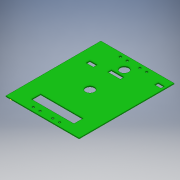
# Autodesk Inventor part: Aquila-2018-Under
Saved by Autodesk Inventor 2018 (Build 220112000, 112)
## iProperties
Created: 2018-08-01
Part Number: Aquila-2018-Under
Material: 一般
Document SubType Name: Modeling
Designer: shun2
Density: 1 g/cm^3
Appearance: 濃い緑
Author: shun2
Autodesk Inventor part; units mm, degrees
ref_plane "YZ Plane" through (0, 0, 0) normal (1, 0, 0) x (0, 1, 0)
ref_plane "XZ Plane" through (0, 0, 0) normal (0, 1, 0) x (-1, 0, 0)
ref_plane "XY Plane" through (0, 0, 0) normal (0, 0, 1) x (1, 0, 0)
sketch "スケッチ4" plane through (0, 0, 0) normal (0, 0, 1) x (1, 0, 0)
  circle A0 centre (127.58, 175.805) radius 0.35
  circle A1 centre (23.4696, 144.78) radius 0.6604
  circle A2 centre (18.4404, 144.78) radius 0.6604
  circle A3 centre (100.9396, 26.035) radius 0.6604
  circle A4 centre (95.9104, 26.035) radius 0.6604
  circle A5 centre (63.105, 150.54) radius 0.6
  circle A6 centre (65.645, 150.54) radius 0.6
  circle A7 centre (68.185, 150.54) radius 0.6
  circle A8 centre (89.59, 26.34) radius 0.6
  circle A9 centre (87.05, 26.34) radius 0.6
  circle A10 centre (84.51, 26.34) radius 0.6
  circle A11 centre (62.96, 25.555) radius 0.508
  circle A12 centre (65.5, 25.555) radius 0.508
  circle A13 centre (68.04, 25.555) radius 0.508
  circle A14 centre (70.58, 25.555) radius 0.508
  circle A15 centre (60.42, 25.555) radius 0.508
  circle A16 centre (75.66, 25.555) radius 0.508
  circle A17 centre (57.88, 25.555) radius 0.508
  circle A18 centre (55.34, 25.555) radius 0.508
  circle A19 centre (78.2, 25.555) radius 0.508
  circle A20 centre (52.8, 25.555) radius 0.508
  circle A21 centre (73.12, 25.555) radius 0.508
  circle A22 centre (50.26, 25.555) radius 0.508
  circle A23 centre (47.72, 25.555) radius 0.508
  circle A24 centre (129.08, 175.805) radius 0.35
  circle A25 centre (130.58, 175.805) radius 0.35
  circle A26 centre (132.08, 175.805) radius 0.35
  circle A27 centre (133.58, 175.805) radius 0.35
  circle A28 centre (124.58, 175.805) radius 0.35
  circle A29 centre (126.08, 175.805) radius 0.35
  circle A30 centre (38, 8) radius 2.15
  circle A31 centre (52, 8) radius 2.15
  circle A32 centre (92, 8) radius 2.15
  circle A33 centre (92, 186.7239) radius 2.15
  circle A34 centre (78, 8) radius 2.15
  circle A35 centre (52, 186.7215) radius 2.15
  circle A36 centre (38, 186.7239) radius 2.15
  circle A37 centre (78, 186.7215) radius 2.15
  line L0 (58.919, 174.3601) -> (58.7286, 174.1804)
  line L1 (58.7286, 174.1804) -> (58.5435, 173.9953)
  line L2 (58.5435, 173.9953) -> (58.3638, 173.8049)
  line L3 (58.3638, 173.8049) -> (58.1897, 173.6093)
  line L4 (58.1897, 173.6093) -> (58.0215, 173.4087)
  line L5 (58.0215, 173.4087) -> (57.8591, 173.2034)
  line L6 (57.8591, 173.2034) -> (57.7027, 172.9933)
  line L7 (57.7027, 172.9933) -> (57.5525, 172.7789)
  line L8 (57.5525, 172.7789) -> (57.4087, 172.5601)
  line L9 (57.4087, 172.5601) -> (57.2712, 172.3373)
  line L10 (57.2712, 172.3373) -> (57.1403, 172.1105)
  line L11 (57.1403, 172.1105) -> (57.0161, 171.8801)
  line L12 (57.0161, 171.8801) -> (56.8986, 171.6461)
  line L13 (56.8986, 171.6461) -> (56.7879, 171.4088)
  line L14 (56.7879, 171.4088) -> (56.6842, 171.1684)
  line L15 (56.6842, 171.1684) -> (56.5875, 170.9251)
  line L16 (56.5875, 170.9251) -> (56.498, 170.6791)
  line L17 (56.498, 170.6791) -> (56.4156, 170.4306)
  line L18 (56.4156, 170.4306) -> (56.3406, 170.1797)
  line L19 (56.3406, 170.1797) -> (56.2728, 169.9268)
  line L20 (56.2728, 169.9268) -> (56.2124, 169.6721)
  line L21 (56.2124, 169.6721) -> (56.1595, 169.4157)
  line L22 (56.1595, 169.4157) -> (56.114, 169.1578)
  line L23 (56.114, 169.1578) -> (56.0761, 168.8988)
  line L24 (56.0761, 168.8988) -> (56.0457, 168.6387)
  line L25 (56.0457, 168.6387) -> (56.0228, 168.3779)
  line L26 (56.0228, 168.3779) -> (56.0076, 168.1165)
  line L27 (56.0076, 168.1165) -> (56, 167.8548)
  line L28 (56, 167.8548) -> (56, 167.593)
  line L29 (56, 167.593) -> (56.0076, 167.3313)
  line L30 (56.0076, 167.3313) -> (56.0228, 167.0699)
  line L31 (56.0228, 167.0699) -> (56.0457, 166.8091)
  line L32 (56.0457, 166.8091) -> (56.0761, 166.5491)
  line L33 (56.0761, 166.5491) -> (56.114, 166.29)
  line L34 (56.114, 166.29) -> (56.1595, 166.0322)
  line L35 (56.1595, 166.0322) -> (56.2124, 165.7758)
  line L36 (56.2124, 165.7758) -> (56.2728, 165.521)
  line L37 (56.2728, 165.521) -> (56.3406, 165.2681)
  line L38 (56.3406, 165.2681) -> (56.4156, 165.0173)
  line L39 (56.4156, 165.0173) -> (56.498, 164.7688)
  line L40 (56.498, 164.7688) -> (56.5875, 164.5227)
  line L41 (56.5875, 164.5227) -> (56.6842, 164.2794)
  line L42 (56.6842, 164.2794) -> (56.7879, 164.039)
  line L43 (56.7879, 164.039) -> (56.8986, 163.8017)
  line L44 (56.8986, 163.8017) -> (57.0161, 163.5677)
  line L45 (57.0161, 163.5677) -> (57.1403, 163.3373)
  line L46 (57.1403, 163.3373) -> (57.2712, 163.1105)
  line L47 (57.2712, 163.1105) -> (57.4087, 162.8877)
  line L48 (57.4087, 162.8877) -> (57.5525, 162.669)
  line L49 (57.5525, 162.669) -> (57.7027, 162.4545)
  line L50 (57.7027, 162.4545) -> (57.8591, 162.2445)
  line L51 (57.8591, 162.2445) -> (58.0215, 162.0391)
  line L52 (58.0215, 162.0391) -> (58.1897, 161.8385)
  line L53 (58.1897, 161.8385) -> (58.3638, 161.643)
  line L54 (58.3638, 161.643) -> (58.5435, 161.4525)
  line L55 (58.5435, 161.4525) -> (58.7286, 161.2674)
  line L56 (58.7286, 161.2674) -> (58.919, 161.0877)
  line L57 (58.919, 161.0877) -> (59.1146, 160.9137)
  line L58 (59.1146, 160.9137) -> (59.3152, 160.7454)
  line L59 (59.3152, 160.7454) -> (59.5206, 160.583)
  line L60 (59.5206, 160.583) -> (59.7306, 160.4266)
  line L61 (59.7306, 160.4266) -> (59.945, 160.2765)
  line L62 (59.945, 160.2765) -> (60.1638, 160.1326)
  line L63 (60.1638, 160.1326) -> (60.3866, 159.9951)
  line L64 (60.3866, 159.9951) -> (60.6134, 159.8642)
  line L65 (60.6134, 159.8642) -> (60.8438, 159.74)
  line L66 (60.8438, 159.74) -> (61.0778, 159.6225)
  line L67 (61.0778, 159.6225) -> (61.3151, 159.5118)
  line L68 (69.1562, 89.378) -> (69.3866, 89.5023)
  line L69 (61.5555, 159.4081) -> (61.7988, 159.3115)
  line L70 (61.7988, 159.3115) -> (62.0448, 159.2219)
  line L71 (62.0448, 159.2219) -> (62.2934, 159.1396)
  line L72 (62.2934, 159.1396) -> (62.5442, 159.0645)
  line L73 (62.5442, 159.0645) -> (62.7971, 158.9967)
  line L74 (62.7971, 158.9967) -> (63.0518, 158.9363)
  line L75 (63.0518, 158.9363) -> (63.3082, 158.8834)
  line L76 (63.3082, 158.8834) -> (63.5661, 158.8379)
  line L77 (63.5661, 158.8379) -> (63.8251, 158.8)
  line L78 (63.8251, 158.8) -> (64.0852, 158.7696)
  line L79 (64.0852, 158.7696) -> (64.346, 158.7468)
  line L80 (64.346, 158.7468) -> (64.6074, 158.7315)
  line L81 (64.6074, 158.7315) -> (64.8691, 158.7239)
  line L82 (64.8691, 158.7239) -> (65.1309, 158.7239)
  line L83 (65.1309, 158.7239) -> (65.3926, 158.7315)
  line L84 (65.3926, 158.7315) -> (65.654, 158.7468)
  line L85 (65.654, 158.7468) -> (65.9148, 158.7696)
  line L86 (65.9148, 158.7696) -> (66.1749, 158.8)
  line L87 (66.1749, 158.8) -> (66.4339, 158.8379)
  line L88 (66.4339, 158.8379) -> (66.6918, 158.8834)
  line L89 (66.6918, 158.8834) -> (66.9482, 158.9363)
  line L90 (66.9482, 158.9363) -> (67.2029, 158.9967)
  line L91 (67.2029, 158.9967) -> (67.4558, 159.0645)
  line L92 (67.4558, 159.0645) -> (67.7066, 159.1396)
  line L93 (67.7066, 159.1396) -> (67.9552, 159.2219)
  line L94 (67.9552, 159.2219) -> (68.2012, 159.3115)
  line L95 (68.2012, 159.3115) -> (68.4445, 159.4081)
  line L96 (68.4445, 159.4081) -> (68.6849, 159.5118)
  line L97 (68.6849, 159.5118) -> (68.9222, 159.6225)
  line L98 (68.9222, 159.6225) -> (69.1562, 159.74)
  line L99 (69.1562, 159.74) -> (69.3866, 159.8642)
  line L100 (69.3866, 159.8642) -> (69.6134, 159.9951)
  line L101 (69.6134, 159.9951) -> (69.8362, 160.1326)
  line L102 (69.8362, 160.1326) -> (70.055, 160.2765)
  line L103 (70.055, 160.2765) -> (70.2694, 160.4266)
  line L104 (70.2694, 160.4266) -> (70.4794, 160.583)
  line L105 (70.4794, 160.583) -> (70.6848, 160.7454)
  line L106 (70.6848, 160.7454) -> (70.8854, 160.9137)
  line L107 (70.8854, 160.9137) -> (71.081, 161.0877)
  line L108 (71.081, 161.0877) -> (71.2714, 161.2674)
  line L109 (71.2714, 161.2674) -> (71.4565, 161.4525)
  line L110 (71.4565, 161.4525) -> (71.6362, 161.643)
  line L111 (71.6362, 161.643) -> (71.8103, 161.8385)
  line L112 (71.8103, 161.8385) -> (71.9785, 162.0391)
  line L113 (71.9785, 162.0391) -> (72.1409, 162.2445)
  line L114 (72.1409, 162.2445) -> (72.2973, 162.4545)
  line L115 (72.2973, 162.4545) -> (72.4475, 162.669)
  line L116 (72.4475, 162.669) -> (72.5913, 162.8877)
  line L117 (72.5913, 162.8877) -> (72.7288, 163.1105)
  line L118 (72.7288, 163.1105) -> (72.8597, 163.3373)
  line L119 (72.8597, 163.3373) -> (72.9839, 163.5677)
  line L120 (72.9839, 163.5677) -> (73.1014, 163.8017)
  line L121 (73.1014, 163.8017) -> (73.2121, 164.039)
  line L122 (73.2121, 164.039) -> (73.3158, 164.2794)
  line L123 (73.3158, 164.2794) -> (73.4125, 164.5227)
  line L124 (73.4125, 164.5227) -> (73.502, 164.7688)
  line L125 (73.502, 164.7688) -> (73.5844, 165.0173)
  line L126 (73.5844, 165.0173) -> (73.6595, 165.2681)
  line L127 (73.6595, 165.2681) -> (73.7272, 165.521)
  line L128 (73.7272, 165.521) -> (73.7876, 165.7758)
  line L129 (73.7876, 165.7758) -> (73.8405, 166.0322)
  line L130 (73.8405, 166.0322) -> (73.886, 166.29)
  line L131 (73.886, 166.29) -> (73.9239, 166.5491)
  line L132 (73.9239, 166.5491) -> (73.9543, 166.8091)
  line L133 (73.9543, 166.8091) -> (73.9772, 167.0699)
  line L134 (73.9772, 167.0699) -> (73.9924, 167.3313)
  line L135 (73.9924, 167.3313) -> (74, 167.593)
  line L136 (57.7027, 102.6314) -> (57.5525, 102.4169)
  line L137 (74, 97.2311) -> (74, 97.4929)
  line L138 (74, 97.4929) -> (73.9924, 97.7546)
  line L139 (73.9924, 97.7546) -> (73.9772, 98.016)
  line L140 (73.9772, 98.016) -> (73.9543, 98.2768)
  line L141 (73.9543, 98.2768) -> (73.9239, 98.5368)
  line L142 (73.9239, 98.5368) -> (73.886, 98.7959)
  line L143 (73.886, 98.7959) -> (73.8405, 99.0537)
  line L144 (73.8405, 99.0537) -> (73.7876, 99.3101)
  line L145 (73.7876, 99.3101) -> (73.7272, 99.5649)
  line L146 (73.7272, 99.5649) -> (73.6595, 99.8178)
  line L147 (73.6595, 99.8178) -> (73.5844, 100.0686)
  line L148 (73.5844, 100.0686) -> (73.502, 100.3171)
  line L149 (73.502, 100.3171) -> (73.4125, 100.5632)
  line L150 (73.4125, 100.5632) -> (73.3158, 100.8065)
  line L151 (73.3158, 100.8065) -> (73.2121, 101.0469)
  line L152 (73.2121, 101.0469) -> (73.1014, 101.2842)
  line L153 (73.1014, 101.2842) -> (72.9839, 101.5181)
  line L154 (61.3151, 159.5118) -> (61.5555, 159.4081)
  line L155 (72.9839, 101.5181) -> (72.8597, 101.7486)
  line L156 (72.8597, 101.7486) -> (72.7288, 101.9753)
  line L157 (72.7288, 101.9753) -> (72.5913, 102.1982)
  line L158 (72.5913, 102.1982) -> (72.4475, 102.4169)
  line L159 (72.4475, 102.4169) -> (72.2973, 102.6314)
  line L160 (72.2973, 102.6314) -> (72.1409, 102.8414)
  line L161 (72.1409, 102.8414) -> (71.9785, 103.0468)
  line L162 (71.9785, 103.0468) -> (71.8103, 103.2473)
  line L163 (71.8103, 103.2473) -> (71.6362, 103.4429)
  line L164 (71.6362, 103.4429) -> (71.4565, 103.6334)
  line L165 (71.4565, 103.6334) -> (71.2714, 103.8185)
  line L166 (71.2714, 103.8185) -> (71.081, 103.9982)
  line L167 (71.081, 103.9982) -> (70.8854, 104.1722)
  line L168 (70.8854, 104.1722) -> (70.6848, 104.3405)
  line L169 (70.6848, 104.3405) -> (70.4794, 104.5029)
  line L170 (70.4794, 104.5029) -> (70.2694, 104.6592)
  line L171 (70.2694, 104.6592) -> (70.055, 104.8094)
  line L172 (70.055, 104.8094) -> (69.8362, 104.9533)
  line L173 (69.8362, 104.9533) -> (69.6134, 105.0907)
  line L174 (69.6134, 105.0907) -> (69.3866, 105.2216)
  line L175 (69.3866, 105.2216) -> (69.1562, 105.3459)
  line L176 (69.1562, 105.3459) -> (68.9222, 105.4634)
  line L177 (68.9222, 105.4634) -> (68.6849, 105.5741)
  line L178 (68.6849, 105.5741) -> (68.4445, 105.6778)
  line L179 (68.4445, 105.6778) -> (68.2012, 105.7744)
  line L180 (68.2012, 105.7744) -> (67.9552, 105.864)
  line L181 (67.9552, 105.864) -> (67.7066, 105.9463)
  line L182 (67.7066, 105.9463) -> (67.4558, 106.0214)
  line L183 (67.4558, 106.0214) -> (67.2029, 106.0892)
  line L184 (67.2029, 106.0892) -> (66.9482, 106.1496)
  line L185 (66.9482, 106.1496) -> (66.6918, 106.2025)
  line L186 (66.6918, 106.2025) -> (66.4339, 106.248)
  line L187 (66.4339, 106.248) -> (66.1749, 106.2859)
  line L188 (66.1749, 106.2859) -> (65.9148, 106.3163)
  line L189 (65.9148, 106.3163) -> (65.654, 106.3391)
  line L190 (65.654, 106.3391) -> (65.3926, 106.3543)
  line L191 (65.3926, 106.3543) -> (65.1309, 106.362)
  line L192 (65.1309, 106.362) -> (64.8691, 106.362)
  line L193 (64.8691, 106.362) -> (64.6074, 106.3543)
  line L194 (64.6074, 106.3543) -> (64.346, 106.3391)
  line L195 (64.346, 106.3391) -> (64.0852, 106.3163)
  line L196 (64.0852, 106.3163) -> (63.8251, 106.2859)
  line L197 (63.8251, 106.2859) -> (63.5661, 106.248)
  line L198 (63.5661, 106.248) -> (63.3082, 106.2025)
  line L199 (63.3082, 106.2025) -> (63.0518, 106.1496)
  line L200 (63.0518, 106.1496) -> (62.7971, 106.0892)
  line L201 (62.7971, 106.0892) -> (62.5442, 106.0214)
  line L202 (62.5442, 106.0214) -> (62.2934, 105.9463)
  line L203 (62.2934, 105.9463) -> (62.0448, 105.864)
  line L204 (62.0448, 105.864) -> (61.7988, 105.7744)
  line L205 (61.7988, 105.7744) -> (61.5555, 105.6778)
  line L206 (61.5555, 105.6778) -> (61.3151, 105.5741)
  line L207 (61.3151, 105.5741) -> (61.0778, 105.4634)
  line L208 (61.0778, 105.4634) -> (60.8438, 105.3459)
  line L209 (60.8438, 105.3459) -> (60.6134, 105.2216)
  line L210 (60.6134, 105.2216) -> (60.3866, 105.0907)
  line L211 (60.3866, 105.0907) -> (60.1638, 104.9533)
  line L212 (60.1638, 104.9533) -> (59.945, 104.8094)
  line L213 (59.945, 104.8094) -> (59.7306, 104.6592)
  line L214 (59.7306, 104.6592) -> (59.5206, 104.5029)
  line L215 (59.5206, 104.5029) -> (59.3152, 104.3405)
  line L216 (59.3152, 104.3405) -> (59.1146, 104.1722)
  line L217 (59.1146, 104.1722) -> (58.919, 103.9982)
  line L218 (58.919, 103.9982) -> (58.7286, 103.8185)
  line L219 (58.7286, 103.8185) -> (58.5435, 103.6334)
  line L220 (58.5435, 103.6334) -> (58.3638, 103.4429)
  line L221 (58.3638, 103.4429) -> (58.1897, 103.2473)
  line L222 (58.1897, 103.2473) -> (58.0215, 103.0468)
  line L223 (58.0215, 103.0468) -> (57.8591, 102.8414)
  line L224 (57.8591, 102.8414) -> (57.7027, 102.6314)
  line L225 (57.5525, 102.4169) -> (57.4087, 102.1982)
  line L226 (57.4087, 102.1982) -> (57.2712, 101.9753)
  line L227 (57.2712, 101.9753) -> (57.1403, 101.7486)
  line L228 (57.1403, 101.7486) -> (57.0161, 101.5181)
  line L229 (57.0161, 101.5181) -> (56.8986, 101.2842)
  line L230 (56.8986, 101.2842) -> (56.7879, 101.0469)
  line L231 (56.7879, 101.0469) -> (56.6842, 100.8065)
  line L232 (56.6842, 100.8065) -> (56.5875, 100.5632)
  line L233 (56.5875, 100.5632) -> (56.498, 100.3171)
  line L234 (56.498, 100.3171) -> (56.4156, 100.0686)
  line L235 (56.4156, 100.0686) -> (56.3406, 99.8178)
  line L236 (56.3406, 99.8178) -> (56.2728, 99.5649)
  line L237 (56.2728, 99.5649) -> (56.2124, 99.3101)
  line L238 (56.2124, 99.3101) -> (56.1595, 99.0537)
  line L239 (56.1595, 99.0537) -> (56.114, 98.7959)
  line L240 (56.114, 98.7959) -> (56.0761, 98.5368)
  line L241 (56.0761, 98.5368) -> (56.0457, 98.2768)
  line L242 (56.0457, 98.2768) -> (56.0228, 98.016)
  line L243 (56.0228, 98.016) -> (56.0076, 97.7546)
  line L244 (56.0076, 97.7546) -> (56, 97.4929)
  line L245 (56, 97.4929) -> (56, 97.2311)
  line L246 (56, 97.2311) -> (56.0076, 96.9693)
  line L247 (56.0076, 96.9693) -> (56.0228, 96.708)
  line L248 (56.0228, 96.708) -> (56.0457, 96.4471)
  line L249 (56.0457, 96.4471) -> (56.0761, 96.1871)
  line L250 (56.0761, 96.1871) -> (56.114, 95.928)
  line L251 (56.114, 95.928) -> (56.1595, 95.6702)
  line L252 (56.1595, 95.6702) -> (56.2124, 95.4138)
  line L253 (56.2124, 95.4138) -> (56.2728, 95.159)
  line L254 (56.2728, 95.159) -> (56.3406, 94.9061)
  line L255 (56.3406, 94.9061) -> (56.4156, 94.6553)
  line L256 (56.4156, 94.6553) -> (56.498, 94.4068)
  line L257 (56.498, 94.4068) -> (56.5875, 94.1608)
  line L258 (56.5875, 94.1608) -> (56.6842, 93.9174)
  line L259 (56.6842, 93.9174) -> (56.7879, 93.677)
  line L260 (56.7879, 93.677) -> (56.8986, 93.4398)
  line L261 (56.8986, 93.4398) -> (57.0161, 93.2058)
  line L262 (57.0161, 93.2058) -> (57.1403, 92.9753)
  line L263 (57.1403, 92.9753) -> (57.2712, 92.7486)
  line L264 (57.2712, 92.7486) -> (57.4087, 92.5258)
  line L265 (57.4087, 92.5258) -> (57.5525, 92.307)
  line L266 (57.5525, 92.307) -> (57.7027, 92.0925)
  line L267 (57.7027, 92.0925) -> (57.8591, 91.8825)
  line L268 (57.8591, 91.8825) -> (58.0215, 91.6772)
  line L269 (58.0215, 91.6772) -> (58.1897, 91.4766)
  line L270 (58.1897, 91.4766) -> (58.3638, 91.281)
  line L271 (58.3638, 91.281) -> (58.5435, 91.0906)
  line L272 (58.5435, 91.0906) -> (58.7286, 90.9054)
  line L273 (58.7286, 90.9054) -> (58.919, 90.7258)
  line L274 (58.919, 90.7258) -> (59.1146, 90.5517)
  line L275 (59.1146, 90.5517) -> (59.3152, 90.3834)
  line L276 (59.3152, 90.3834) -> (59.5206, 90.221)
  line L277 (59.5206, 90.221) -> (59.7306, 90.0647)
  line L278 (59.7306, 90.0647) -> (59.945, 89.9145)
  line L279 (59.945, 89.9145) -> (60.1638, 89.7706)
  line L280 (60.1638, 89.7706) -> (60.3866, 89.6332)
  line L281 (60.3866, 89.6332) -> (60.6134, 89.5023)
  line L282 (60.6134, 89.5023) -> (60.8438, 89.378)
  line L283 (60.8438, 89.378) -> (61.0778, 89.2605)
  line L284 (61.0778, 89.2605) -> (61.3151, 89.1499)
  line L285 (61.3151, 89.1499) -> (61.5555, 89.0462)
  line L286 (61.5555, 89.0462) -> (61.7988, 88.9495)
  line L287 (61.7988, 88.9495) -> (62.0448, 88.86)
  line L288 (62.0448, 88.86) -> (62.2934, 88.7776)
  line L289 (62.2934, 88.7776) -> (62.5442, 88.7025)
  line L290 (62.5442, 88.7025) -> (62.7971, 88.6347)
  line L291 (62.7971, 88.6347) -> (63.0518, 88.5744)
  line L292 (63.0518, 88.5744) -> (63.3082, 88.5214)
  line L293 (63.3082, 88.5214) -> (63.5661, 88.476)
  line L294 (63.5661, 88.476) -> (63.8251, 88.438)
  line L295 (63.8251, 88.438) -> (64.0852, 88.4076)
  line L296 (64.0852, 88.4076) -> (64.346, 88.3848)
  line L297 (64.346, 88.3848) -> (64.6074, 88.3696)
  line L298 (64.6074, 88.3696) -> (64.8691, 88.362)
  line L299 (64.8691, 88.362) -> (65.1309, 88.362)
  line L300 (65.1309, 88.362) -> (65.3926, 88.3696)
  line L301 (65.3926, 88.3696) -> (65.654, 88.3848)
  line L302 (65.654, 88.3848) -> (65.9148, 88.4076)
  line L303 (65.9148, 88.4076) -> (66.1749, 88.438)
  line L304 (66.1749, 88.438) -> (66.4339, 88.476)
  line L305 (66.4339, 88.476) -> (66.6918, 88.5214)
  line L306 (66.6918, 88.5214) -> (66.9482, 88.5744)
  line L307 (66.9482, 88.5744) -> (67.2029, 88.6347)
  line L308 (67.2029, 88.6347) -> (67.4558, 88.7025)
  line L309 (67.4558, 88.7025) -> (67.7066, 88.7776)
  line L310 (67.7066, 88.7776) -> (67.9552, 88.86)
  line L311 (67.9552, 88.86) -> (68.2012, 88.9495)
  line L312 (68.2012, 88.9495) -> (68.4445, 89.0462)
  line L313 (68.4445, 89.0462) -> (68.6849, 89.1499)
  line L314 (68.6849, 89.1499) -> (68.9222, 89.2605)
  line L315 (68.9222, 89.2605) -> (69.1562, 89.378)
  line L316 (69.3866, 89.5023) -> (69.6134, 89.6332)
  line L317 (69.6134, 89.6332) -> (69.8362, 89.7706)
  line L318 (69.8362, 89.7706) -> (70.055, 89.9145)
  line L319 (70.055, 89.9145) -> (70.2694, 90.0647)
  line L320 (70.2694, 90.0647) -> (70.4794, 90.221)
  line L321 (70.4794, 90.221) -> (70.6848, 90.3834)
  line L322 (70.6848, 90.3834) -> (70.8854, 90.5517)
  line L323 (70.8854, 90.5517) -> (71.081, 90.7258)
  line L324 (71.081, 90.7258) -> (71.2714, 90.9054)
  line L325 (71.2714, 90.9054) -> (71.4565, 91.0906)
  line L326 (71.4565, 91.0906) -> (71.6362, 91.281)
  line L327 (71.6362, 91.281) -> (71.8103, 91.4766)
  line L328 (71.8103, 91.4766) -> (71.9785, 91.6772)
  line L329 (71.9785, 91.6772) -> (72.1409, 91.8825)
  line L330 (72.1409, 91.8825) -> (72.2973, 92.0925)
  line L331 (72.2973, 92.0925) -> (72.4475, 92.307)
  line L332 (72.4475, 92.307) -> (72.5913, 92.5258)
  line L333 (72.5913, 92.5258) -> (72.7288, 92.7486)
  line L334 (72.7288, 92.7486) -> (72.8597, 92.9753)
  line L335 (72.8597, 92.9753) -> (72.9839, 93.2058)
  line L336 (72.9839, 93.2058) -> (73.1014, 93.4398)
  line L337 (73.1014, 93.4398) -> (73.2121, 93.677)
  line L338 (73.2121, 93.677) -> (73.3158, 93.9174)
  line L339 (73.3158, 93.9174) -> (73.4125, 94.1608)
  line L340 (64.6074, 176.7163) -> (64.346, 176.7011)
  line L341 (73.4125, 94.1608) -> (73.502, 94.4068)
  line L342 (73.502, 94.4068) -> (73.5844, 94.6553)
  line L343 (73.5844, 94.6553) -> (73.6595, 94.9061)
  line L344 (73.6595, 94.9061) -> (73.7272, 95.159)
  line L345 (73.7272, 95.159) -> (73.7876, 95.4138)
  line L346 (73.7876, 95.4138) -> (73.8405, 95.6702)
  line L347 (73.8405, 95.6702) -> (73.886, 95.928)
  line L348 (73.886, 95.928) -> (73.9239, 96.1871)
  line L349 (73.9239, 96.1871) -> (73.9543, 96.4471)
  line L350 (73.9543, 96.4471) -> (73.9772, 96.708)
  line L351 (73.9772, 96.708) -> (73.9924, 96.9693)
  line L352 (73.9924, 96.9693) -> (74, 97.2311)
  line L353 (74, 167.593) -> (74, 167.8548)
  line L354 (74, 167.8548) -> (73.9924, 168.1165)
  line L355 (73.9924, 168.1165) -> (73.9772, 168.3779)
  line L356 (73.9772, 168.3779) -> (73.9543, 168.6387)
  line L357 (73.9543, 168.6387) -> (73.9239, 168.8988)
  line L358 (73.9239, 168.8988) -> (73.886, 169.1578)
  line L359 (73.886, 169.1578) -> (73.8405, 169.4157)
  line L360 (73.8405, 169.4157) -> (73.7876, 169.6721)
  line L361 (73.7876, 169.6721) -> (73.7272, 169.9268)
  line L362 (73.7272, 169.9268) -> (73.6595, 170.1797)
  line L363 (73.6595, 170.1797) -> (73.5844, 170.4306)
  line L364 (73.5844, 170.4306) -> (73.502, 170.6791)
  line L365 (73.502, 170.6791) -> (73.4125, 170.9251)
  line L366 (73.4125, 170.9251) -> (73.3158, 171.1684)
  line L367 (73.3158, 171.1684) -> (73.2121, 171.4088)
  line L368 (73.2121, 171.4088) -> (73.1014, 171.6461)
  line L369 (73.1014, 171.6461) -> (72.9839, 171.8801)
  line L370 (72.9839, 171.8801) -> (72.8597, 172.1105)
  line L371 (72.8597, 172.1105) -> (72.7288, 172.3373)
  line L372 (72.7288, 172.3373) -> (72.5913, 172.5601)
  line L373 (72.5913, 172.5601) -> (72.4475, 172.7789)
  line L374 (72.4475, 172.7789) -> (72.2973, 172.9933)
  line L375 (72.2973, 172.9933) -> (72.1409, 173.2034)
  line L376 (72.1409, 173.2034) -> (71.9785, 173.4087)
  line L377 (71.9785, 173.4087) -> (71.8103, 173.6093)
  line L378 (71.8103, 173.6093) -> (71.6362, 173.8049)
  line L379 (71.6362, 173.8049) -> (71.4565, 173.9953)
  line L380 (71.4565, 173.9953) -> (71.2714, 174.1804)
  line L381 (71.2714, 174.1804) -> (71.081, 174.3601)
  line L382 (71.081, 174.3601) -> (70.8854, 174.5342)
  line L383 (70.8854, 174.5342) -> (70.6848, 174.7025)
  line L384 (70.6848, 174.7025) -> (70.4794, 174.8649)
  line L385 (70.4794, 174.8649) -> (70.2694, 175.0212)
  line L386 (70.2694, 175.0212) -> (70.055, 175.1714)
  line L387 (70.055, 175.1714) -> (69.8362, 175.3152)
  line L388 (69.8362, 175.3152) -> (69.6134, 175.4527)
  line L389 (69.6134, 175.4527) -> (69.3866, 175.5836)
  line L390 (69.3866, 175.5836) -> (69.1562, 175.7079)
  line L391 (69.1562, 175.7079) -> (68.9222, 175.8254)
  line L392 (68.9222, 175.8254) -> (68.6849, 175.936)
  line L393 (68.6849, 175.936) -> (68.4445, 176.0397)
  line L394 (68.4445, 176.0397) -> (68.2012, 176.1364)
  line L395 (68.2012, 176.1364) -> (67.9552, 176.2259)
  line L396 (67.9552, 176.2259) -> (67.7066, 176.3083)
  line L397 (67.7066, 176.3083) -> (67.4558, 176.3834)
  line L398 (67.4558, 176.3834) -> (67.2029, 176.4511)
  line L399 (67.2029, 176.4511) -> (66.9482, 176.5115)
  line L400 (66.9482, 176.5115) -> (66.6918, 176.5645)
  line L401 (66.6918, 176.5645) -> (66.4339, 176.6099)
  line L402 (66.4339, 176.6099) -> (66.1749, 176.6479)
  line L403 (66.1749, 176.6479) -> (65.9148, 176.6783)
  line L404 (65.9148, 176.6783) -> (65.654, 176.7011)
  line L405 (65.654, 176.7011) -> (65.3926, 176.7163)
  line L406 (65.3926, 176.7163) -> (65.1309, 176.7239)
  line L407 (65.1309, 176.7239) -> (64.8691, 176.7239)
  line L408 (64.8691, 176.7239) -> (64.6074, 176.7163)
  line L409 (64.346, 176.7011) -> (64.0852, 176.6783)
  line L410 (64.0852, 176.6783) -> (63.8251, 176.6479)
  line L411 (63.8251, 176.6479) -> (63.5661, 176.6099)
  line L412 (63.5661, 176.6099) -> (63.3082, 176.5645)
  line L413 (63.3082, 176.5645) -> (63.0518, 176.5115)
  line L414 (63.0518, 176.5115) -> (62.7971, 176.4511)
  line L415 (62.7971, 176.4511) -> (62.5442, 176.3834)
  line L416 (62.5442, 176.3834) -> (62.2934, 176.3083)
  line L417 (62.2934, 176.3083) -> (62.0448, 176.2259)
  line L418 (62.0448, 176.2259) -> (61.7988, 176.1364)
  line L419 (61.7988, 176.1364) -> (61.5555, 176.0397)
  line L420 (61.5555, 176.0397) -> (61.3151, 175.936)
  line L421 (61.3151, 175.936) -> (61.0778, 175.8254)
  line L422 (61.0778, 175.8254) -> (60.8438, 175.7079)
  line L423 (60.8438, 175.7079) -> (60.6134, 175.5836)
  line L424 (60.6134, 175.5836) -> (60.3866, 175.4527)
  line L425 (60.3866, 175.4527) -> (60.1638, 175.3152)
  line L426 (60.1638, 175.3152) -> (59.945, 175.1714)
  line L427 (59.945, 175.1714) -> (59.7306, 175.0212)
  line L428 (59.7306, 175.0212) -> (59.5206, 174.8649)
  line L429 (59.5206, 174.8649) -> (59.3152, 174.7025)
  line L430 (59.3152, 174.7025) -> (59.1146, 174.5342)
  line L431 (59.1146, 174.5342) -> (58.919, 174.3601)
  line L432 (-10, 194.7239) -> (-10, 0)
  line L433 (140, 194.7239) -> (-10, 194.7239)
  line L434 (140, 0) -> (140, 194.7239)
  line L435 (-10, 0) -> (140, 0)
  line L436 (78, 146.5788) -> (52, 146.5788)
  line L437 (-10, 194.7239) -> (140, 194.7239)
  line L438 (140, 0) -> (-10, 0)
  line L439 (-10, 194.7239) -> (-10, 0)
  line L440 (140, 194.7239) -> (140, 0)
  line L441 (52, 154.1355) -> (78, 154.1355)
  line L442 (52, 154.1355) -> (52, 146.5788)
  line L443 (78, 154.1355) -> (78, 146.5788)
  line L444 (22.1852, 20.07) -> (109.3416, 20.07)
  line L445 (109.3416, 20.07) -> (109.3416, 38.9202)
  line L446 (109.3416, 38.9202) -> (22.1852, 38.9202)
  line L447 (22.1852, 38.9202) -> (22.1852, 20.07)
  circle A38 centre (38, 8) radius 2.15
  circle A39 centre (52, 8) radius 2.15
  circle A40 centre (78, 8) radius 2.15
  circle A41 centre (92, 8) radius 2.15
  circle A42 centre (65, 97.362) radius 9
  circle A43 centre (65, 167.7239) radius 9
  circle A44 centre (38, 186.7239) radius 2.15
  circle A45 centre (52, 186.7215) radius 2.15
  circle A46 centre (78, 186.7215) radius 2.15
  circle A47 centre (92, 186.7239) radius 2.15
  line L448 (13.6863, 148.4905) -> (28.6396, 148.4905)
  line L449 (28.6396, 148.4905) -> (28.6396, 140.4912)
  line L450 (28.6396, 140.4912) -> (13.6863, 140.4912)
  line L451 (13.6863, 140.4912) -> (13.6863, 148.4905)
  line L452 (122.8325, 179.5316) -> (135.5762, 179.5316)
  line L453 (135.5762, 179.5316) -> (135.5762, 172.1105)
  line L454 (135.5762, 172.1105) -> (122.8325, 172.1105)
  line L455 (122.8325, 172.1105) -> (122.8325, 179.5316)
  point P0 (0, 0)
  constraints: 912 end point, 48 centre point, 8 coincident, 8 concentric, 8 equal length, 6 perpendicular, 6 tangent, 4 horizontal
sketch "スケッチ5" plane through (0, 0, 0) normal (0, 0, 1) x (1, 0, 0)
  point P0 (0, 0)
extrude "押し出し4" add sketch "スケッチ4" along normal blind 1.8 contours L433 L434 L435 L432
